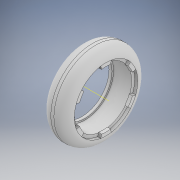
# Autodesk Inventor part: PrednjiKotač_635z_lezaj_v.2.0
Saved by Autodesk Inventor 2020 (Build 240168000, 168)
## iProperties
Created: 2020-10-01
Part Number: PrednjiKotač_635z_lezaj_v.2.0
Material: Generic
Document SubType Name: Modeling
Designer: Sičaja
Density: 1 g/cm^3
Appearance: Default
Author: Sičaja
Autodesk Inventor part; units mm, degrees
ref_plane "YZ Plane" through (0, 0, 0) normal (1, 0, 0) x (0, 1, 0)
ref_plane "XZ Plane" through (0, 0, 0) normal (0, 1, 0) x (-1, 0, 0)
ref_plane "XY Plane" through (0, 0, 0) normal (0, 0, 1) x (1, 0, 0)
sketch "Sketch1" plane through (0, 0, 0) normal (1, 0, 0) x (0, 1, 0)
  circle A0 centre (0, 0) radius 13.75
  circle A1 centre (0, 0) radius 9.5
  circle A2 centre (0, 0) radius 2.5
  circle A3 centre (0, 0) radius 10.5
  dimension "d0" = 27.5
  dimension "d1" = 19
  dimension "d2" = 5
  dimension "d3" = 21
  constraints: 4 centre point, 4 coincident
  measures "d0" diameter of A0
  measures "d1" diameter of A1
  measures "d2" diameter of A2
  measures "d3" diameter of A3
sketch "Sketch2" plane through (0, 0, 0) normal (1, 0, 0) x (0, 1, 0)
  circle A0 centre (0, 0) radius 13.75 projected
  circle A1 centre (0, 0) radius 10.5 projected
extrude "Extrusion1" add sketch "Sketch1" along normal mid plane 6 contours A3
extrude "Extrusion2" add sketch "Sketch2" along normal mid plane 8
fillet "Fillet1" radius 3.5 2 edges at (4, -13.75, 0) (-4, -13.75, 0)
sketch "Sketch3" plane through (-3, 0, 0) normal (-1, 0, 0) x (0, 0, 1)
  circle A0 centre (0, 0) radius 9
  circle A1 centre (0, 0) radius 10.5
  circle A2 centre (0, 0) radius 10.5143
  dimension "d9" = 18
  constraints: 3 centre point, 3 coincident
  measures "d9" diameter of A0
extrude "Extrusion3" add sketch "Sketch3" along normal blind 1 contours A1 | A2
sketch "Sketch4" plane through (3, 0, 0) normal (1, 0, 0) x (0, 0, -1)
  circle A0 centre (0, 0) radius 10.5 projected
  circle A1 centre (0, 0) radius 10.5 projected
  circle A2 centre (0, 0) radius 10.5
  circle A3 centre (0, 0) radius 10
  line L0 (1.7444, -10.3541) -> (1.6211, -9.8677)
  line L1 (0, -10.5) -> (0, -10)
  line L2 (-1.6211, -9.8677) -> (-1.7444, -10.3541)
  circle A4 centre (0, 0) radius 10.5 projected
  circle A5 centre (0, 0) radius 9.4
  line L3 (1.7444, -10.3541) -> (1.4732, -9.2838)
  line L4 (-1.7444, -10.3541) -> (-1.4732, -9.2838)
  dimension "d18" = 20
  dimension "d19" = 18.8
  constraints: 10 end point, 6 point on circle, 3 coincident, 2 centre point, 1 vertical alignment, 2 other
  measures "d18" diameter of A3
  measures "d19" diameter of A5
extrude "Extrusion4" add sketch "Sketch4" along normal blind 1 contours L2 A3 L1 A0 | A0 L1 A3 L0 | L4 A5 L3 A3 picked at (0, -9.5914)
draft "FaceDraft2" angle 5 pull direction (1, 0, 0) faces at (3.6667, -9.3986, 0.1644) fixed edges at (4, -9.4, 0)
pattern_circular "Circular Pattern1" count 6 over 360 about axis through (3, 0, 0) along (-1, 0, 0) of "Extrusion4", "FaceDraft2"
body "Solid1"
